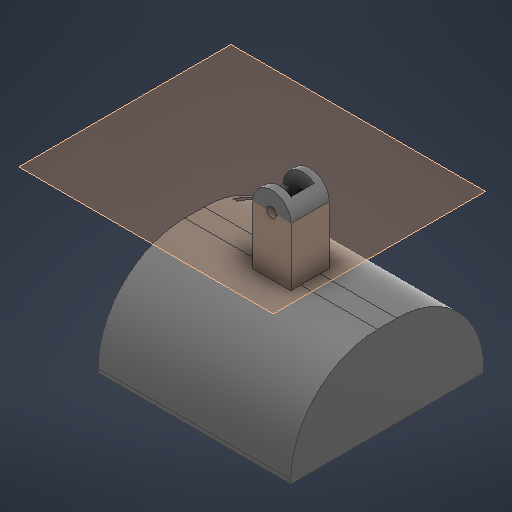
# Autodesk Inventor part: BuddyRobotBase
Saved by Autodesk Inventor 2026.2 (Build 302298000, 298)
## iProperties
Created: 2026-09-15
Part Number: BuddyRobotBase
Material: Generic
Document SubType Name: Modeling
Designer: User
Density: 1 g/cm^3
Appearance: Default
Author: User
Autodesk Inventor part; units mm, degrees
(part 1 of 2)
ref_plane "YZ Plane" through (0, 0, 0) normal (1, 0, 0) x (0, 1, 0)
ref_plane "XZ Plane" through (0, 0, 0) normal (0, 1, 0) x (-1, 0, 0)
ref_plane "XY Plane" through (0, 0, 0) normal (0, 0, 1) x (1, 0, 0)
sketch "Sketch1" plane through (0, 0, 0) normal (0, 1, 0) x (-1, 0, 0)
  line L0 (50, 50) -> (-50, 50)
  line L1 (-50, 50) -> (-50, -50)
  line L2 (-50, -50) -> (50, -50)
  line L3 (50, -50) -> (50, 50)
  line L4 (50, 50) -> (-50, -50) construction
  line L5 (-50, 50) -> (50, -50) construction
  point P0 (0, 0)
  dimension "d1" = 100
  dimension "d2" = 100
  constraints: 12 end point, 2 midpoint, 2 parallel, 1 horizontal, 1 perpendicular
  measures "d1" distance of L0.end L1.end
  measures "d2" distance of L0.start L0.end
extrude "Base" add sketch "Sketch1" along normal blind 2
sketch "Sketch2" plane through (50, 0, 50) normal (1, 0, 0) x (0, 0, -1)
  line L0 (0, 2) -> (100, 2) projected
  line L1 (0, 2) -> (100, 2)
  arc A0 (45, 47) -> (0, 2) centre (45, 2) ccw
  line L2 (0, 0) -> (0, 2) projected
  arc A1 (100, 2) -> (55, 47) centre (55, 2) ccw
  line L3 (100, 0) -> (100, 2) projected
  line L4 (45, 47) -> (55, 47)
  point P0 (50, 0)
  dimension "d6" = 10
  constraints: 4 end point, 4 point on circle, 3 tangent, 2 centre point, 1 collinear, 1 equal radius, 1 horizontal, 1 horizontal alignment
  measures "d6" distance of L4.start L4.end
extrude "Box" add sketch "Sketch2" against normal blind 100
shell "Shell" thickness 2 removed faces 1 at (-50, 15.6667, -1.6667)
sketch "Sketch4" plane through (50, 0, -50) normal (0, 0, -1) x (-1, 0, 0)
  line L0 (0, 2) -> (100, 2) projected
  line L1 (96, 2) -> (98, 2)
  line L2 (98, 2) -> (98, 45)
  line L3 (98, 45) -> (96, 45)
  line L4 (96, 45) -> (96, 2)
  line L5 (0, 47) -> (100, 47) projected
  line L6 (100, 2) -> (100, 47) projected
  point P0 (50, 0)
  dimension "d10" = 2
  dimension "d11" = 2
  dimension "d12" = 2
  constraints: 8 end point, 2 parallel, 1 horizontal, 1 perpendicular, 1 point on line
  measures "d10" distance between parallel lines of L5 L3
  measures "d11" distance between parallel lines of L6 L2
  measures "d12" distance between parallel lines of L2 L4
extrude "DoorSlot" cut sketch "Sketch4" against normal up to next
sketch "Sketch6" plane through (50, 47, 5) normal (0, 1, 0) x (1, 0, 0)
  line L0 (-40, 14.9) -> (-60, 14.9)
  line L1 (-60, 14.9) -> (-60, -4.9)
  line L2 (-60, -4.9) -> (-40, -4.9)
  line L3 (-40, -4.9) -> (-40, 14.9)
  line L4 (-40, 14.9) -> (-60, -4.9) construction
  line L5 (-60, 14.9) -> (-40, -4.9) construction
  line L6 (0, 10) -> (0, 0) projected
  point P0 (-50, 5)
  point P1 (-50, 5)
  dimension "d18" = 20
  dimension "d19" = 19.8
  dimension "d20" = 40
  constraints: 12 end point, 2 midpoint, 2 parallel, 1 coincident, 1 horizontal, 1 perpendicular
  measures "d18" distance of L0.start L0.end
  measures "d19" distance of L0.end L1.end
  measures "d20" distance between parallel lines of L6 L3
extrude "Extrusion5" add sketch "Sketch6" along normal blind 30 and the other way blind 0.5
sketch "Sketch7" plane through (-10, 46.7324, 9.9) normal (0, 0, 1) x (1, 0, 0)
  line L0 (0, 30.2676) -> (20, 30.2676) projected
  circle A0 centre (10, 30.2676) radius 10
  line L1 (20, 0) -> (20, 30.2676) projected
  point P0 (10, -46.7324)
  point P1 (20, 30.2676)
  point P2 (0, 30.2676)
  constraints: 1 centre point, 1 midpoint, 1 tangent
extrude "Extrusion6" add sketch "Sketch7" against normal blind 19.8 contours A0 L0 picked at (12.78, 34.8248)
sketch "Sketch8" plane through (-10, 46.7324, 9.9) normal (0, 0, 1) x (1, 0, 0)
  arc A0 (20, 30.2676) -> (0, 30.2676) centre (10, 30.2676) ccw projected
  circle A1 centre (10, 30.2676) radius 2.5
  point P0 (10, -46.7324)
  dimension "d27" = 5
  constraints: 1 centre point, 1 coincident
  measures "d27" diameter of A1
extrude "Extrusion7" cut sketch "Sketch8" against normal up to next
sketch "Sketch9" plane through (-50, 45, 5) normal (0, -1, 0) x (1, 0, 0)
  point P0 (50, -5)
ref_plane "Work Plane1" through (-10, 77, -9.9) normal (0, 1, 0) x (0, 0, 1)
sketch "Sketch10" plane through (-10, 77, -9.9) normal (0, 1, 0) x (0, 0, 1)
  line L0 (3.8, 16) -> (15.8, 16)
  line L1 (15.8, 16) -> (15.8, 4)
  line L2 (15.8, 4) -> (3.8, 4)
  line L3 (3.8, 4) -> (3.8, 16)
  line L4 (3.8, 16) -> (15.8, 4) construction
  line L5 (15.8, 16) -> (3.8, 4) construction
  line L6 (0, 0) -> (19.8, 0) projected
  line L7 (19.8, 0) -> (19.8, 20) projected
  point P0 (9.9, 10)
  point P1 (9.8, 10)
  dimension "d31" = 4
  dimension "d32" = 4
  dimension "d33" = 12
  dimension "d34" = 12
  constraints: 12 end point, 2 midpoint, 2 parallel, 1 horizontal, 1 perpendicular
  measures "d31" distance between parallel lines of L6 L2
  measures "d32" distance between parallel lines of L7 L1
  measures "d33" distance of L0.end L1.end
  measures "d34" distance of L1.end L2.end
extrude "Extrusion8" cut sketch "Sketch10" along normal blind 20 and the other way blind 40
sketch "Sketch11" plane through (-10, 47, -5) normal (-1, 0, 0) x (0, 0, 1)
  line L0 (-1.1, 38) -> (10.9, 38) projected
  line L1 (10.9, 32.5) -> (10.9, 27.5) projected
  line L2 (-1.1, 38) -> (10.9, 38)
  line L3 (10.9, 38) -> (10.9, 30)
  line L4 (10.9, 30) -> (-1.1, 30)
  line L5 (-1.1, 30) -> (-1.1, 38)
  point P0 (5, -47)
  point P1 (10.9, 32.5)
  point P2 (10.9, 38)
  constraints: 8 end point, 2 parallel, 1 horizontal, 1 midpoint, 1 perpendicular
extrude "Extrusion9" cut sketch "Sketch11" against normal up to next
sketch "Sketch12" plane through (48, 2, -48) normal (-1, 0, 0) x (0, 0, 1)
  arc A0 (43, 43) -> (0, 0) centre (43, 0) ccw projected
  line L0 (1.179, 10) -> (94.821, 10) construction
  line L1 (96, 0) -> (0, 0) projected
  arc A1 (96, 0) -> (53, 43) centre (53, 0) ccw projected
  spline S0 degree 2 poles (10.9376, 10.1) (10.3824, 9.8828) (9.5169, 9.8828) knots 0 0 0 1 1 1
  spline S1 degree 2 poles (9.5169, 9.8828) (9.41, 9.8828) (9.2203, 10.0828) (9.2203, 10.1897) knots 0 0 0 1 2 2 2
  line L2 (9.2203, 10.1897) -> (9.2203, 10.9103)
  spline S2 degree 2 poles (9.2203, 10.9103) (9.2203, 11.2621) (9.2652, 11.9172) knots 0 0 0 1 1 1
  spline S3 degree 2 poles (9.2652, 11.9172) (9.3134, 12.6241) (9.3169, 12.9414) knots 0 0 0 1 1 1
  spline S4 degree 2 poles (9.3169, 12.9414) (9.3169, 13.169) (9.3445, 13.6207) knots 0 0 0 1 1 1
  spline S5 degree 2 poles (9.3445, 13.6207) (9.3617, 13.7414) (9.4272, 13.7828) knots 0 0 0 1 1 1
  spline S6 degree 2 poles (9.4272, 13.7828) (9.7617, 13.8862) (10.1893, 13.8862) knots 0 0 0 1 1 1
  spline S7 degree 2 poles (10.1893, 13.8862) (10.6272, 13.8862) (11.0272, 13.5897) knots 0 0 0 1 1 1
  spline S8 degree 2 poles (11.0272, 13.5897) (11.4893, 13.2483) (11.4893, 12.7448) knots 0 0 0 1 1 1
  spline S9 degree 2 poles (11.4893, 12.7448) (11.4893, 12.1103) (10.9962, 11.7448) knots 0 0 0 1 1 1
  spline S10 degree 2 poles (10.9962, 11.7448) (11.3652, 11.5862) (11.7341, 11.2) (11.7341, 10.9724) knots 0 0 0 1 2 2 2
  spline S11 degree 2 poles (11.7341, 10.9724) (11.7341, 10.6724) (11.41, 10.3931) knots 0 0 0 1 1 1
  spline S12 degree 2 poles (11.41, 10.3931) (11.1858, 10.1966) (10.9376, 10.1) knots 0 0 0 1 1 1
  spline S13 degree 2 poles (10.1927, 13.3828) (9.9238, 13.3828) (9.8134, 13.3655) knots 0 0 0 1 1 1
  line L3 (9.8134, 13.3655) -> (9.81, 12.931)
  line L4 (9.81, 12.931) -> (9.7583, 11.9724)
  spline S14 degree 2 poles (9.7583, 11.9724) (10.11, 11.9414) (10.1341, 11.9448) knots 0 0 0 1 1 1
  spline S15 degree 2 poles (10.1341, 11.9448) (10.5065, 11.9759) (10.7445, 12.1793) knots 0 0 0 1 1 1
  spline S16 degree 2 poles (10.7445, 12.1793) (10.9996, 12.4) (10.9996, 12.7448) knots 0 0 0 1 1 1
  spline S17 degree 2 poles (10.9996, 12.7448) (10.9996, 12.9828) (10.4824, 13.3828) (10.1927, 13.3828) knots 0 0 0 1 2 2 2
  line L5 (10.4686, 11.4) -> (10.2065, 11.4414)
  spline S18 degree 2 poles (10.2065, 11.4414) (10.1755, 11.4414) (10.0445, 11.4345) (10.01, 11.4345) knots 0 0 0 1 2 2 2
  spline S19 degree 2 poles (10.01, 11.4345) (9.8755, 11.4345) (9.7238, 11.4552) knots 0 0 0 1 1 1
  spline S20 degree 2 poles (9.7238, 11.4552) (9.71, 11.1448) (9.71, 10.9) knots 0 0 0 1 1 1
  line L6 (9.71, 10.9) -> (9.71, 10.3897)
  spline S21 degree 2 poles (9.71, 10.3897) (10.3583, 10.4103) (10.7652, 10.5724) knots 0 0 0 1 1 1
  spline S22 degree 2 poles (10.7652, 10.5724) (10.9376, 10.6379) (11.0962, 10.7793) knots 0 0 0 1 1 1
  spline S23 degree 2 poles (11.0962, 10.7793) (11.2479, 10.9069) (11.2479, 10.9724) knots 0 0 0 1 1 1
  spline S24 degree 2 poles (11.2479, 10.9724) (11.2479, 11.0897) (10.9307, 11.2345) knots 0 0 0 1 1 1
  spline S25 degree 2 poles (10.9307, 11.2345) (10.6927, 11.3448) (10.4686, 11.4) knots 0 0 0 1 1 1
  spline S26 degree 2 poles (14.3031, 11.4448) (14.3031, 11.2655) (14.3065, 10.5552) (14.3065, 10.3759) knots 0 0 0 1 2 2 2
  spline S27 degree 2 poles (14.3065, 10.3759) (14.3065, 10.3241) (14.3238, 10.1) (14.3238, 10.0448) knots 0 0 0 1 2 2 2
  spline S28 degree 2 poles (14.3238, 10.0448) (14.3238, 9.9379) (14.179, 9.8034) (14.0755, 9.8034) knots 0 0 0 1 2 2 2
  spline S29 degree 2 poles (14.0755, 9.8034) (13.8858, 9.8034) (13.8341, 10.0379) knots 0 0 0 1 1 1
  spline S30 degree 2 poles (13.8341, 10.0379) (13.5238, 9.8759) (13.1203, 9.8759) knots 0 0 0 1 1 1
  spline S31 degree 2 poles (13.1203, 9.8759) (12.7962, 9.8759) (12.5824, 10.0207) knots 0 0 0 1 1 1
  spline S32 degree 2 poles (12.5824, 10.0207) (12.3479, 10.1793) (12.3031, 10.4828) knots 0 0 0 1 1 1
  spline S33 degree 2 poles (12.3031, 10.4828) (12.21, 11.1379) (12.21, 11.6517) knots 0 0 0 1 1 1
  spline S34 degree 2 poles (12.21, 11.6517) (12.21, 11.9897) (12.2824, 12.4241) knots 0 0 0 1 1 1
  spline S35 degree 2 poles (12.2824, 12.4241) (12.3169, 12.6379) (12.5169, 12.6379) knots 0 0 0 1 1 1
  spline S36 degree 2 poles (12.5169, 12.6379) (12.6238, 12.6379) (12.7652, 12.5034) (12.7652, 12.3966) knots 0 0 0 1 2 2 2
  spline S37 degree 2 poles (12.7652, 12.3966) (12.7652, 12.2828) (12.6962, 11.7828) (12.6962, 11.6517) knots 0 0 0 1 2 2 2
  spline S38 degree 2 poles (12.6962, 11.6517) (12.6962, 11.2379) (12.7514, 10.6483) (12.8031, 10.4724) knots 0 0 0 1 2 2 2
  spline S39 degree 2 poles (12.8031, 10.4724) (12.8858, 10.4276) (13.0445, 10.3793) (13.1203, 10.3793) knots 0 0 0 1 2 2 2
  spline S40 degree 2 poles (13.1203, 10.3793) (13.4548, 10.3793) (13.8238, 10.4862) knots 0 0 0 1 1 1
  line L7 (13.8238, 10.4862) -> (13.8203, 10.9862)
  line L8 (13.8203, 10.9862) -> (13.8169, 11.4655)
  spline S41 degree 2 poles (13.8169, 11.4655) (13.8169, 12) (13.8617, 12.3931) knots 0 0 0 1 1 1
  spline S42 degree 2 poles (13.8617, 12.3931) (13.8893, 12.6207) (14.0996, 12.6207) knots 0 0 0 1 1 1
  spline S43 degree 2 poles (14.0996, 12.6207) (14.2065, 12.6207) (14.3479, 12.4828) (14.3445, 12.3793) knots 0 0 0 1 2 2 2
  line L9 (14.3445, 12.3793) -> (14.3031, 11.4448)
  spline S44 degree 2 poles (17.1996, 12.1828) (17.1686, 11.8207) (17.1686, 11.4552) knots 0 0 0 1 1 1
  spline S45 degree 2 poles (17.1686, 11.4552) (17.1686, 10.631) (17.2445, 10.2103) knots 0 0 0 1 1 1
  spline S46 degree 2 poles (17.2445, 10.2103) (17.2514, 10.1759) (17.2514, 10.1552) knots 0 0 0 1 1 1
  spline S47 degree 2 poles (17.2514, 10.1552) (17.2514, 10.0552) (17.1134, 9.9276) (17.0203, 9.9276) knots 0 0 0 1 2 2 2
  spline S48 degree 2 poles (17.0203, 9.9276) (16.8686, 9.9276) (16.7962, 10.1517) knots 0 0 0 1 1 1
  spline S49 degree 2 poles (16.7962, 10.1517) (16.6169, 10.0207) (16.2341, 9.8862) (16.0272, 9.8862) knots 0 0 0 1 2 2 2
  spline S50 degree 2 poles (16.0272, 9.8862) (15.5134, 9.8862) (15.179, 10.2276) knots 0 0 0 1 1 1
  spline S51 degree 2 poles (15.179, 10.2276) (14.8307, 10.5759) (14.8307, 11.1241) knots 0 0 0 1 1 1
  spline S52 degree 2 poles (14.8307, 11.1241) (14.8307, 11.7828) (15.5307, 12.5793) (16.0893, 12.5793) knots 0 0 0 1 2 2 2
  spline S53 degree 2 poles (16.0893, 12.5793) (16.3755, 12.5793) (16.5341, 12.4897) knots 0 0 0 1 1 1
  line L10 (16.5341, 12.4897) -> (16.7652, 12.3207)
  spline S54 degree 2 poles (16.7652, 12.3207) (16.7996, 13.3621) (16.8479, 13.7207) knots 0 0 0 1 1 1
  spline S55 degree 2 poles (16.8479, 13.7207) (16.879, 13.9414) (17.0721, 13.9414) knots 0 0 0 1 1 1
  spline S56 degree 2 poles (17.0721, 13.9414) (17.2962, 13.9414) (17.2962, 13.7) knots 0 0 0 1 1 1
  spline S57 degree 2 poles (17.2962, 13.7) (17.2962, 13.3586) (17.1996, 12.1828) knots 0 0 0 1 1 1
  spline S58 degree 2 poles (16.0996, 12.1207) (15.6858, 12.1207) (15.2686, 11.6276) (15.2686, 11.1345) knots 0 0 0 1 2 2 2
  spline S59 degree 2 poles (15.2686, 11.1345) (15.2686, 10.8138) (15.7203, 10.3552) (16.0272, 10.3552) knots 0 0 0 1 2 2 2
  spline S60 degree 2 poles (16.0272, 10.3552) (16.2341, 10.3552) (16.379, 10.431) knots 0 0 0 1 1 1
  spline S61 degree 2 poles (16.379, 10.431) (16.4617, 10.4759) (16.6514, 10.6379) knots 0 0 0 1 1 1
  spline S62 degree 2 poles (16.6514, 10.6379) (16.6893, 10.669) (16.7238, 10.7138) knots 0 0 0 1 1 1
  line L11 (16.7238, 10.7138) -> (16.7169, 11.1414)
  line L12 (16.7169, 11.1414) -> (16.7203, 11.4276)
  line L13 (16.7203, 11.4276) -> (16.7238, 11.7207)
  spline S63 degree 2 poles (16.7238, 11.7207) (16.6307, 11.9207) (16.3169, 12.1207) (16.0996, 12.1207) knots 0 0 0 1 2 2 2
  spline S64 degree 2 poles (20.1755, 12.1828) (20.1445, 11.8207) (20.1445, 11.4552) knots 0 0 0 1 1 1
  spline S65 degree 2 poles (20.1445, 11.4552) (20.1445, 10.631) (20.2203, 10.2103) knots 0 0 0 1 1 1
  spline S66 degree 2 poles (20.2203, 10.2103) (20.2272, 10.1759) (20.2272, 10.1552) knots 0 0 0 1 1 1
  spline S67 degree 2 poles (20.2272, 10.1552) (20.2272, 10.0552) (20.0893, 9.9276) (19.9962, 9.9276) knots 0 0 0 1 2 2 2
  spline S68 degree 2 poles (19.9962, 9.9276) (19.8445, 9.9276) (19.7721, 10.1517) knots 0 0 0 1 1 1
  spline S69 degree 2 poles (19.7721, 10.1517) (19.5927, 10.0207) (19.21, 9.8862) (19.0031, 9.8862) knots 0 0 0 1 2 2 2
  spline S70 degree 2 poles (19.0031, 9.8862) (18.4893, 9.8862) (18.1548, 10.2276) knots 0 0 0 1 1 1
  spline S71 degree 2 poles (18.1548, 10.2276) (17.8065, 10.5759) (17.8065, 11.1241) knots 0 0 0 1 1 1
  spline S72 degree 2 poles (17.8065, 11.1241) (17.8065, 11.7828) (18.5065, 12.5793) (19.0652, 12.5793) knots 0 0 0 1 2 2 2
  spline S73 degree 2 poles (19.0652, 12.5793) (19.3514, 12.5793) (19.51, 12.4897) knots 0 0 0 1 1 1
  line L14 (19.51, 12.4897) -> (19.741, 12.3207)
  spline S74 degree 2 poles (19.741, 12.3207) (19.7755, 13.3621) (19.8238, 13.7207) knots 0 0 0 1 1 1
  spline S75 degree 2 poles (19.8238, 13.7207) (19.8548, 13.9414) (20.0479, 13.9414) knots 0 0 0 1 1 1
  spline S76 degree 2 poles (20.0479, 13.9414) (20.2721, 13.9414) (20.2721, 13.7) knots 0 0 0 1 1 1
  spline S77 degree 2 poles (20.2721, 13.7) (20.2721, 13.3586) (20.1755, 12.1828) knots 0 0 0 1 1 1
  spline S78 degree 2 poles (19.0755, 12.1207) (18.6617, 12.1207) (18.2445, 11.6276) (18.2445, 11.1345) knots 0 0 0 1 2 2 2
  spline S79 degree 2 poles (18.2445, 11.1345) (18.2445, 10.8138) (18.6962, 10.3552) (19.0031, 10.3552) knots 0 0 0 1 2 2 2
  spline S80 degree 2 poles (19.0031, 10.3552) (19.21, 10.3552) (19.3548, 10.431) knots 0 0 0 1 1 1
  spline S81 degree 2 poles (19.3548, 10.431) (19.4376, 10.4759) (19.6272, 10.6379) knots 0 0 0 1 1 1
  spline S82 degree 2 poles (19.6272, 10.6379) (19.6652, 10.669) (19.6996, 10.7138) knots 0 0 0 1 1 1
  line L15 (19.6996, 10.7138) -> (19.6927, 11.1414)
  line L16 (19.6927, 11.1414) -> (19.6962, 11.4276)
  line L17 (19.6962, 11.4276) -> (19.6996, 11.7207)
  spline S83 degree 2 poles (19.6996, 11.7207) (19.6065, 11.9207) (19.2927, 12.1207) (19.0755, 12.1207) knots 0 0 0 1 2 2 2
  line L18 (23.0272, 12.2069) -> (22.1721, 10.3552)
  spline S84 degree 2 poles (22.1721, 10.3552) (21.8548, 9.6793) (21.6858, 9.2241) knots 0 0 0 1 1 1
  line L19 (21.6858, 9.2241) -> (21.5238, 8.7448)
  spline S85 degree 2 poles (21.5238, 8.7448) (21.4583, 8.569) (21.3031, 8.569) knots 0 0 0 1 1 1
  spline S86 degree 2 poles (21.3031, 8.569) (21.1996, 8.569) (21.0479, 8.7034) (21.0479, 8.8069) knots 0 0 0 1 2 2 2
  spline S87 degree 2 poles (21.0479, 8.8069) (21.0479, 9.0517) (21.5824, 10.2379) knots 0 0 0 1 1 1
  line L20 (21.5824, 10.2379) -> (20.6962, 11.9414)
  line L21 (20.6962, 11.9414) -> (20.5824, 12.1207)
  spline S88 degree 2 poles (20.5824, 12.1207) (20.5169, 12.2345) (20.5169, 12.3138) knots 0 0 0 1 1 1
  spline S89 degree 2 poles (20.5169, 12.3138) (20.5169, 12.4138) (20.6721, 12.569) (20.7686, 12.569) knots 0 0 0 1 2 2 2
  spline S90 degree 2 poles (20.7686, 12.569) (20.8824, 12.569) (20.9445, 12.4793) knots 0 0 0 1 1 1
  spline S91 degree 2 poles (20.9445, 12.4793) (21.3652, 11.8931) (21.8479, 10.8103) knots 0 0 0 1 1 1
  line L22 (21.8479, 10.8103) -> (22.2169, 11.6724)
  spline S92 degree 2 poles (22.2169, 11.6724) (22.4134, 12.1138) (22.5962, 12.4345) knots 0 0 0 1 1 1
  spline S93 degree 2 poles (22.5962, 12.4345) (22.6755, 12.5724) (22.8031, 12.5724) knots 0 0 0 1 1 1
  spline S94 degree 2 poles (22.8031, 12.5724) (22.9031, 12.5724) (23.0583, 12.4276) (23.0583, 12.331) knots 0 0 0 1 2 2 2
  spline S95 degree 2 poles (23.0583, 12.331) (23.0583, 12.2759) (23.0272, 12.2069) knots 0 0 0 1 1 1
  spline S96 degree 2 poles (26.8686, 10.1) (26.3134, 9.8828) (25.4479, 9.8828) knots 0 0 0 1 1 1
  spline S97 degree 2 poles (25.4479, 9.8828) (25.341, 9.8828) (25.1514, 10.0828) (25.1514, 10.1897) knots 0 0 0 1 2 2 2
  line L23 (25.1514, 10.1897) -> (25.1514, 10.9103)
  spline S98 degree 2 poles (25.1514, 10.9103) (25.1514, 11.2621) (25.1962, 11.9172) knots 0 0 0 1 1 1
  spline S99 degree 2 poles (25.1962, 11.9172) (25.2445, 12.6241) (25.2479, 12.9414) knots 0 0 0 1 1 1
  spline S100 degree 2 poles (25.2479, 12.9414) (25.2479, 13.169) (25.2755, 13.6207) knots 0 0 0 1 1 1
  spline S101 degree 2 poles (25.2755, 13.6207) (25.2927, 13.7414) (25.3583, 13.7828) knots 0 0 0 1 1 1
  spline S102 degree 2 poles (25.3583, 13.7828) (25.6927, 13.8862) (26.1203, 13.8862) knots 0 0 0 1 1 1
  spline S103 degree 2 poles (26.1203, 13.8862) (26.5583, 13.8862) (26.9583, 13.5897) knots 0 0 0 1 1 1
  spline S104 degree 2 poles (26.9583, 13.5897) (27.4203, 13.2483) (27.4203, 12.7448) knots 0 0 0 1 1 1
  spline S105 degree 2 poles (27.4203, 12.7448) (27.4203, 12.1103) (26.9272, 11.7448) knots 0 0 0 1 1 1
  spline S106 degree 2 poles (26.9272, 11.7448) (27.2962, 11.5862) (27.6652, 11.2) (27.6652, 10.9724) knots 0 0 0 1 2 2 2
  spline S107 degree 2 poles (27.6652, 10.9724) (27.6652, 10.6724) (27.341, 10.3931) knots 0 0 0 1 1 1
  spline S108 degree 2 poles (27.341, 10.3931) (27.1169, 10.1966) (26.8686, 10.1) knots 0 0 0 1 1 1
  spline S109 degree 2 poles (26.1238, 13.3828) (25.8548, 13.3828) (25.7445, 13.3655) knots 0 0 0 1 1 1
  line L24 (25.7445, 13.3655) -> (25.741, 12.931)
  line L25 (25.741, 12.931) -> (25.6893, 11.9724)
  spline S110 degree 2 poles (25.6893, 11.9724) (26.041, 11.9414) (26.0652, 11.9448) knots 0 0 0 1 1 1
  spline S111 degree 2 poles (26.0652, 11.9448) (26.4376, 11.9759) (26.6755, 12.1793) knots 0 0 0 1 1 1
  spline S112 degree 2 poles (26.6755, 12.1793) (26.9307, 12.4) (26.9307, 12.7448) knots 0 0 0 1 1 1
  spline S113 degree 2 poles (26.9307, 12.7448) (26.9307, 12.9828) (26.4134, 13.3828) (26.1238, 13.3828) knots 0 0 0 1 2 2 2
  line L26 (26.3996, 11.4) -> (26.1376, 11.4414)
  spline S114 degree 2 poles (26.1376, 11.4414) (26.1065, 11.4414) (25.9755, 11.4345) (25.941, 11.4345) knots 0 0 0 1 2 2 2
  spline S115 degree 2 poles (25.941, 11.4345) (25.8065, 11.4345) (25.6548, 11.4552) knots 0 0 0 1 1 1
  spline S116 degree 2 poles (25.6548, 11.4552) (25.641, 11.1448) (25.641, 10.9) knots 0 0 0 1 1 1
  line L27 (25.641, 10.9) -> (25.641, 10.3897)
  spline S117 degree 2 poles (25.641, 10.3897) (26.2893, 10.4103) (26.6962, 10.5724) knots 0 0 0 1 1 1
  spline S118 degree 2 poles (26.6962, 10.5724) (26.8686, 10.6379) (27.0272, 10.7793) knots 0 0 0 1 1 1
  spline S119 degree 2 poles (27.0272, 10.7793) (27.179, 10.9069) (27.179, 10.9724) knots 0 0 0 1 1 1
  spline S120 degree 2 poles (27.179, 10.9724) (27.179, 11.0897) (26.8617, 11.2345) knots 0 0 0 1 1 1
  spline S121 degree 2 poles (26.8617, 11.2345) (26.6238, 11.3448) (26.3996, 11.4) knots 0 0 0 1 1 1
  spline S122 degree 2 poles (29.1479, 9.8552) (28.7341, 9.8552) (28.4341, 10.1621) knots 0 0 0 1 1 1
  spline S123 degree 2 poles (28.4341, 10.1621) (28.0996, 10.5034) (28.0824, 11.0793) knots 0 0 0 1 1 1
  spline S124 degree 2 poles (28.0824, 11.0793) (28.0686, 11.6379) (28.3652, 12.0621) knots 0 0 0 1 1 1
  spline S125 degree 2 poles (28.3652, 12.0621) (28.71, 12.5655) (29.3272, 12.5655) knots 0 0 0 1 1 1
  spline S126 degree 2 poles (29.3272, 12.5655) (29.8238, 12.5655) (30.0755, 12.1138) knots 0 0 0 1 1 1
  spline S127 degree 2 poles (30.0755, 12.1138) (30.279, 11.7483) (30.2721, 11.231) knots 0 0 0 1 1 1
  spline S128 degree 2 poles (30.2721, 11.231) (30.2652, 10.6828) (29.9859, 10.2966) knots 0 0 0 1 1 1
  spline S129 degree 2 poles (29.9859, 10.2966) (29.6686, 9.8552) (29.1479, 9.8552) knots 0 0 0 1 1 1
  spline S130 degree 2 poles (29.2962, 12.0621) (28.9341, 12.0655) (28.7307, 11.7172) knots 0 0 0 1 1 1
  spline S131 degree 2 poles (28.7307, 11.7172) (28.5686, 11.4379) (28.5686, 11.0793) knots 0 0 0 1 1 1
  spline S132 degree 2 poles (28.5686, 11.0793) (28.5686, 10.7207) (28.7652, 10.5207) knots 0 0 0 1 1 1
  spline S133 degree 2 poles (28.7652, 10.5207) (28.9272, 10.3552) (29.1479, 10.3552) knots 0 0 0 1 1 1
  spline S134 degree 2 poles (29.1479, 10.3552) (29.4065, 10.3552) (29.5893, 10.5414) knots 0 0 0 1 1 1
  spline S135 degree 2 poles (29.5893, 10.5414) (29.7996, 10.7517) (29.8134, 11.1034) knots 0 0 0 1 1 1
  spline S136 degree 2 poles (29.8134, 11.1034) (29.8479, 12.0586) (29.2962, 12.0621) knots 0 0 0 1 1 1
  spline S137 degree 2 poles (32.5376, 12.1069) (32.4859, 12.1069) (32.3445, 12.1172) (32.2927, 12.1172) knots 0 0 0 1 2 2 2
  spline S138 degree 2 poles (32.2927, 12.1172) (32.2341, 12.1172) (31.9548, 12.0793) knots 0 0 0 1 1 1
  line L28 (31.9548, 12.0793) -> (31.9996, 10.6172)
  line L29 (31.9996, 10.6172) -> (32.0031, 10.5103)
  line L30 (32.0031, 10.5103) -> (32.0065, 10.3828)
  spline S139 degree 2 poles (32.0065, 10.3828) (32.0169, 9.8414) (31.7479, 9.8414) knots 0 0 0 1 1 1
  spline S140 degree 2 poles (31.7479, 9.8414) (31.6479, 9.8414) (31.5031, 9.969) (31.5031, 10.0655) knots 0 0 0 1 2 2 2
  spline S141 degree 2 poles (31.5031, 10.0655) (31.5031, 10.1621) (31.5169, 10.5379) (31.5169, 10.631) knots 0 0 0 1 2 2 2
  line L31 (31.5169, 10.631) -> (31.4686, 12.0759)
  spline S142 degree 2 poles (31.4686, 12.0759) (31.2893, 12.0828) (30.9203, 12.1172) knots 0 0 0 1 1 1
  spline S143 degree 2 poles (30.9203, 12.1172) (30.6996, 12.1483) (30.6996, 12.3621) knots 0 0 0 1 1 1
  spline S144 degree 2 poles (30.6996, 12.3621) (30.6996, 12.4724) (30.8341, 12.6138) (30.9376, 12.6138) knots 0 0 0 1 2 2 2
  line L32 (30.9376, 12.6138) -> (31.4548, 12.5724)
  spline S145 degree 2 poles (31.4548, 12.5724) (31.4548, 12.7) (31.4341, 13.1207) (31.4341, 13.2138) knots 0 0 0 1 2 2 2
  spline S146 degree 2 poles (31.4341, 13.2138) (31.4341, 13.3207) (31.5755, 13.4552) (31.679, 13.4552) knots 0 0 0 1 2 2 2
  spline S147 degree 2 poles (31.679, 13.4552) (31.9031, 13.4552) (31.941, 13.0931) knots 0 0 0 1 1 1
  spline S148 degree 2 poles (31.941, 13.0931) (31.9479, 13) (31.9479, 12.8724) knots 0 0 0 1 1 1
  line L33 (31.9479, 12.8724) -> (31.9445, 12.7276)
  line L34 (31.9445, 12.7276) -> (31.941, 12.5759)
  spline S149 degree 2 poles (31.941, 12.5759) (32.2479, 12.6138) (32.2927, 12.6138) knots 0 0 0 1 1 1
  spline S150 degree 2 poles (32.2927, 12.6138) (32.5479, 12.6138) (32.6272, 12.5897) knots 0 0 0 1 1 1
  spline S151 degree 2 poles (32.6272, 12.5897) (32.779, 12.5414) (32.779, 12.3586) knots 0 0 0 1 1 1
  spline S152 degree 2 poles (32.779, 12.3586) (32.779, 12.2483) (32.6445, 12.1069) (32.5376, 12.1069) knots 0 0 0 1 2 2 2
  spline S153 degree 2 poles (37.6686, 13.3897) (37.5134, 13.1621) (37.4169, 12.9103) knots 0 0 0 1 1 1
  line L35 (37.4169, 12.9103) -> (37.2307, 12.369)
  line L36 (37.2307, 12.369) -> (36.5652, 10.569)
  spline S154 degree 2 poles (36.5652, 10.569) (36.4479, 10.2552) (36.2927, 9.9517) knots 0 0 0 1 1 1
  spline S155 degree 2 poles (36.2927, 9.9517) (36.2134, 9.8034) (36.0686, 9.8034) knots 0 0 0 1 1 1
  spline S156 degree 2 poles (36.0686, 9.8034) (35.879, 9.8034) (35.8031, 9.9966) knots 0 0 0 1 1 1
  spline S157 degree 2 poles (35.8031, 9.9966) (35.5031, 10.7483) (35.1376, 12.1586) knots 0 0 0 1 1 1
  line L37 (35.1376, 12.1586) -> (34.941, 12.8414)
  spline S158 degree 2 poles (34.941, 12.8414) (34.7962, 13.3552) (34.7962, 13.5138) knots 0 0 0 1 1 1
  spline S159 degree 2 poles (34.7962, 13.5138) (34.7962, 13.6241) (34.8755, 13.6966) knots 0 0 0 1 1 1
  spline S160 degree 2 poles (34.8755, 13.6966) (34.9479, 13.7621) (35.0479, 13.7621) knots 0 0 0 1 1 1
  spline S161 degree 2 poles (35.0479, 13.7621) (35.2376, 13.7621) (35.2893, 13.5586) knots 0 0 0 1 1 1
  line L38 (35.2893, 13.5586) -> (35.3824, 13.1276)
  line L39 (35.3824, 13.1276) -> (35.6203, 12.2897)
  spline S162 degree 2 poles (35.6203, 12.2897) (35.8548, 11.369) (36.0824, 10.7034) knots 0 0 0 1 1 1
  line L40 (36.0824, 10.7034) -> (36.0962, 10.7448)
  line L41 (36.0962, 10.7448) -> (36.7583, 12.5379)
  line L42 (36.7583, 12.5379) -> (36.9686, 13.1448)
  spline S163 degree 2 poles (36.9686, 13.1448) (37.11, 13.5103) (37.2686, 13.6966) knots 0 0 0 1 1 1
  spline S164 degree 2 poles (37.2686, 13.6966) (37.3514, 13.7966) (37.4617, 13.7966) knots 0 0 0 1 1 1
  spline S165 degree 2 poles (37.4617, 13.7966) (37.5617, 13.7966) (37.7169, 13.6448) (37.7169, 13.5379) knots 0 0 0 1 2 2 2
  spline S166 degree 2 poles (37.7169, 13.5379) (37.7169, 13.4655) (37.6686, 13.3897) knots 0 0 0 1 1 1
  line L43 (39.4721, 9.9966) -> (38.9824, 9.9966)
  line L44 (38.9824, 9.9966) -> (38.4927, 10)
  spline S167 degree 2 poles (38.4927, 10) (38.3203, 10) (38.2514, 10.0207) knots 0 0 0 1 1 1
  spline S168 degree 2 poles (38.2514, 10.0207) (38.1238, 10.0655) (38.1238, 10.2103) knots 0 0 0 1 1 1
  spline S169 degree 2 poles (38.1238, 10.2103) (38.1238, 10.4586) (38.51, 10.4586) knots 0 0 0 1 1 1
  line L45 (38.51, 10.4586) -> (38.6307, 10.4552)
  line L46 (38.6307, 10.4552) -> (38.7307, 10.4517)
  spline S170 degree 2 poles (38.7307, 10.4517) (38.7307, 10.569) (38.6893, 11.0345) (38.6893, 11.1517) knots 0 0 0 1 2 2 2
  spline S171 degree 2 poles (38.6893, 11.1517) (38.6893, 11.4655) (38.7445, 12.1069) knots 0 0 0 1 1 1
  spline S172 degree 2 poles (38.7445, 12.1069) (38.7996, 12.7345) (38.7962, 13.0621) knots 0 0 0 1 1 1
  spline S173 degree 2 poles (38.7962, 13.0621) (38.4652, 12.8034) (38.3755, 12.8034) knots 0 0 0 1 1 1
  spline S174 degree 2 poles (38.3755, 12.8034) (38.2755, 12.8034) (38.1307, 12.9517) (38.1307, 13.0483) knots 0 0 0 1 2 2 2
  spline S175 degree 2 poles (38.1307, 13.0483) (38.1307, 13.1655) (38.3445, 13.331) knots 0 0 0 1 1 1
  spline S176 degree 2 poles (38.3445, 13.331) (38.4755, 13.4276) (38.7203, 13.6345) knots 0 0 0 1 1 1
  spline S177 degree 2 poles (38.7203, 13.6345) (38.941, 13.8552) (39.1376, 13.8552) knots 0 0 0 1 1 1
  spline S178 degree 2 poles (39.1376, 13.8552) (39.3031, 13.8552) (39.3031, 13.6655) knots 0 0 0 1 1 1
  spline S179 degree 2 poles (39.3031, 13.6655) (39.3031, 13.6069) (39.2721, 13.3828) (39.2721, 13.3241) knots 0 0 0 1 2 2 2
  spline S180 degree 2 poles (39.2721, 13.3241) (39.2721, 13.2448) (39.2893, 12.9138) (39.2893, 12.831) knots 0 0 0 1 2 2 2
  spline S181 degree 2 poles (39.2893, 12.831) (39.2893, 12.5483) (39.1721, 11.431) (39.1721, 11.1517) knots 0 0 0 1 2 2 2
  spline S182 degree 2 poles (39.1721, 11.1517) (39.1721, 11.0069) (39.21, 10.5966) (39.2134, 10.4655) knots 0 0 0 1 2 2 2
  line L47 (39.2134, 10.4655) -> (39.4721, 10.469)
  spline S183 degree 2 poles (39.4721, 10.469) (39.579, 10.469) (39.7134, 10.3345) (39.7134, 10.2345) knots 0 0 0 1 2 2 2
  spline S184 degree 2 poles (39.7134, 10.2345) (39.7134, 10.131) (39.579, 9.9966) (39.4721, 9.9966) knots 0 0 0 1 2 2 2
  spline S185 degree 2 poles (40.6721, 9.769) (40.5445, 9.769) (40.3652, 9.9483) (40.3652, 10.0759) knots 0 0 0 1 2 2 2
  spline S186 degree 2 poles (40.3652, 10.0759) (40.3652, 10.2034) (40.5445, 10.3828) (40.6721, 10.3828) knots 0 0 0 1 2 2 2
  spline S187 degree 2 poles (40.6721, 10.3828) (40.7996, 10.3828) (40.979, 10.2034) (40.979, 10.0759) knots 0 0 0 1 2 2 2
  spline S188 degree 2 poles (40.979, 10.0759) (40.979, 9.9483) (40.7996, 9.769) (40.6721, 9.769) knots 0 0 0 1 2 2 2
  spline S189 degree 2 poles (42.7859, 9.9034) (42.0341, 9.9034) (41.6893, 10.5897) knots 0 0 0 1 1 1
  spline S190 degree 2 poles (41.6893, 10.5897) (41.4272, 11.1207) (41.4272, 11.969) knots 0 0 0 1 1 1
  spline S191 degree 2 poles (41.4272, 11.969) (41.4272, 12.6862) (41.7686, 13.2207) knots 0 0 0 1 1 1
  spline S192 degree 2 poles (41.7686, 13.2207) (42.1721, 13.8448) (42.8617, 13.8448) knots 0 0 0 1 1 1
  spline S193 degree 2 poles (42.8617, 13.8448) (43.5134, 13.8448) (43.8755, 13.2897) knots 0 0 0 1 1 1
  spline S194 degree 2 poles (43.8755, 13.2897) (44.1893, 12.8103) (44.1893, 12.1207) knots 0 0 0 1 1 1
  spline S195 degree 2 poles (44.1893, 12.1207) (44.1893, 11.0138) (43.4893, 9.9034) (42.7859, 9.9034) knots 0 0 0 1 2 2 2
  spline S196 degree 2 poles (42.8617, 13.369) (42.3996, 13.369) (42.1307, 12.9) knots 0 0 0 1 1 1
  spline S197 degree 2 poles (42.1307, 12.9) (41.9065, 12.5103) (41.9065, 12.0103) knots 0 0 0 1 1 1
  spline S198 degree 2 poles (41.9065, 12.0103) (41.9065, 11.1966) (42.3479, 10.3793) (42.7859, 10.3793) knots 0 0 0 1 2 2 2
  spline S199 degree 2 poles (42.7859, 10.3793) (43.31, 10.3793) (43.5376, 10.9793) knots 0 0 0 1 1 1
  spline S200 degree 2 poles (43.5376, 10.9793) (43.6962, 11.3931) (43.6962, 12.031) knots 0 0 0 1 1 1
  spline S201 degree 2 poles (43.6962, 12.031) (43.6962, 12.7) (43.279, 13.369) (42.8617, 13.369) knots 0 0 0 1 2 2 2
  spline S202 degree 2 poles (47.5583, 11.1759) (47.2238, 11.1414) (46.3617, 11.1414) knots 0 0 0 1 1 1
  spline S203 degree 2 poles (46.3617, 11.1414) (46.1548, 11.1414) (46.1548, 11.3345) knots 0 0 0 1 1 1
  spline S204 degree 2 poles (46.1548, 11.3345) (46.1548, 11.5276) (46.3617, 11.5276) knots 0 0 0 1 1 1
  spline S205 degree 2 poles (46.3617, 11.5276) (46.5583, 11.5276) (47.341, 11.5621) (47.5341, 11.5621) knots 0 0 0 1 2 2 2
  spline S206 degree 2 poles (47.5341, 11.5621) (47.7548, 11.5621) (47.7548, 11.369) knots 0 0 0 1 1 1
  spline S207 degree 2 poles (47.7548, 11.369) (47.7548, 11.2) (47.5583, 11.1759) knots 0 0 0 1 1 1
  spline S208 degree 2 poles (52.8721, 13.1241) (52.6893, 13.1241) (52.3065, 13.1552) knots 0 0 0 1 1 1
  spline S209 degree 2 poles (52.3065, 13.1552) (51.9376, 13.1828) (51.7445, 13.1793) knots 0 0 0 1 1 1
  line L48 (51.7445, 13.1793) -> (51.5686, 13.1793)
  spline S210 degree 2 poles (51.5686, 13.1793) (51.5755, 12.8379) (51.6341, 12.069) knots 0 0 0 1 1 1
  spline S211 degree 2 poles (51.6341, 12.069) (51.6893, 11.3552) (51.6893, 10.9586) knots 0 0 0 1 1 1
  spline S212 degree 2 poles (51.6893, 10.9586) (51.6893, 10.8724) (51.7238, 10.5207) (51.7238, 10.431) knots 0 0 0 1 2 2 2
  spline S213 degree 2 poles (51.7238, 10.431) (51.7238, 10.2655) (51.6686, 10.1414) knots 0 0 0 1 1 1
  spline S214 degree 2 poles (51.6686, 10.1414) (51.5996, 9.9793) (51.4548, 9.9793) knots 0 0 0 1 1 1
  spline S215 degree 2 poles (51.4548, 9.9793) (51.3548, 9.9793) (51.1962, 10.1172) (51.1962, 10.2276) knots 0 0 0 1 2 2 2
  spline S216 degree 2 poles (51.1962, 10.2276) (51.1962, 10.2655) (51.2203, 10.4138) (51.2203, 10.4483) knots 0 0 0 1 2 2 2
  spline S217 degree 2 poles (51.2203, 10.4483) (51.2203, 10.5724) (51.1893, 11.0552) (51.1893, 11.1793) knots 0 0 0 1 2 2 2
  spline S218 degree 2 poles (51.1893, 11.1793) (51.1893, 11.5345) (51.1307, 12.1759) knots 0 0 0 1 1 1
  spline S219 degree 2 poles (51.1307, 12.1759) (51.0721, 12.8655) (51.0652, 13.169) knots 0 0 0 1 1 1
  line L49 (51.0652, 13.169) -> (50.841, 13.1655)
  spline S220 degree 2 poles (50.841, 13.1655) (50.2996, 13.1655) (49.9893, 13.2448) knots 0 0 0 1 1 1
  spline S221 degree 2 poles (49.9893, 13.2448) (49.7893, 13.2966) (49.7893, 13.4897) knots 0 0 0 1 1 1
  spline S222 degree 2 poles (49.7893, 13.4897) (49.7893, 13.5931) (49.8548, 13.669) knots 0 0 0 1 1 1
  spline S223 degree 2 poles (49.8548, 13.669) (49.9272, 13.7552) (50.0445, 13.7483) knots 0 0 0 1 1 1
  spline S224 degree 2 poles (50.0445, 13.7483) (50.1307, 13.7448) (50.441, 13.7034) knots 0 0 0 1 1 1
  spline S225 degree 2 poles (50.441, 13.7034) (50.6859, 13.6724) (50.841, 13.6724) knots 0 0 0 1 1 1
  spline S226 degree 2 poles (50.841, 13.6724) (50.9893, 13.6724) (51.5927, 13.6862) (51.741, 13.6862) knots 0 0 0 1 2 2 2
  spline S227 degree 2 poles (51.741, 13.6862) (51.9307, 13.6862) (52.679, 13.631) (52.8721, 13.631) knots 0 0 0 1 2 2 2
  spline S228 degree 2 poles (52.8721, 13.631) (52.9755, 13.631) (53.1203, 13.4862) (53.1203, 13.3759) knots 0 0 0 1 2 2 2
  spline S229 degree 2 poles (53.1203, 13.3759) (53.1203, 13.2724) (52.9755, 13.1241) (52.8721, 13.1241) knots 0 0 0 1 2 2 2
  spline S230 degree 2 poles (55.2203, 9.8345) (55.1755, 9.8345) (55.0514, 9.9448) knots 0 0 0 1 1 1
  spline S231 degree 2 poles (55.0514, 9.9448) (54.941, 10.0448) (54.8859, 10.1241) knots 0 0 0 1 1 1
  spline S232 degree 2 poles (54.8859, 10.1241) (54.6479, 9.9966) (54.2859, 9.8655) (54.1652, 9.8655) knots 0 0 0 1 2 2 2
  spline S233 degree 2 poles (54.1652, 9.8655) (53.5859, 9.8655) (53.3203, 10.1931) knots 0 0 0 1 1 1
  spline S234 degree 2 poles (53.3203, 10.1931) (53.0721, 10.5) (53.0721, 11.131) knots 0 0 0 1 1 1
  spline S235 degree 2 poles (53.0721, 11.131) (53.0721, 11.731) (53.8962, 12.5828) (54.4686, 12.5828) knots 0 0 0 1 2 2 2
  spline S236 degree 2 poles (54.4686, 12.5828) (54.6824, 12.5828) (54.9514, 12.4724) knots 0 0 0 1 1 1
  spline S237 degree 2 poles (54.9514, 12.4724) (55.2859, 12.331) (55.2859, 12.1379) knots 0 0 0 1 1 1
  spline S238 degree 2 poles (55.2859, 12.1379) (55.2859, 12.069) (55.2376, 12.0172) knots 0 0 0 1 1 1
  spline S239 degree 2 poles (55.2376, 12.0172) (55.2134, 11.9241) (55.1859, 11.4931) (55.1824, 11.1552) knots 0 0 0 1 2 2 2
  spline S240 degree 2 poles (55.1824, 11.1552) (55.179, 10.8483) (55.2238, 10.6724) knots 0 0 0 1 1 1
  spline S241 degree 2 poles (55.2238, 10.6724) (55.2479, 10.5621) (55.379, 10.2345) knots 0 0 0 1 1 1
  spline S242 degree 2 poles (55.379, 10.2345) (55.3962, 10.1897) (55.4376, 10.1034) knots 0 0 0 1 1 1
  line L50 (55.4376, 10.1034) -> (55.4514, 10.0621)
  spline S243 degree 2 poles (55.4514, 10.0621) (55.4514, 9.9621) (55.3134, 9.8345) (55.2203, 9.8345) knots 0 0 0 1 2 2 2
  spline S244 degree 2 poles (54.7065, 11.5552) (54.7065, 11.6621) (54.7341, 11.9138) (54.7617, 12.0517) knots 0 0 0 1 2 2 2
  spline S245 degree 2 poles (54.7617, 12.0517) (54.6686, 12.1) (54.5376, 12.1448) (54.4996, 12.1448) knots 0 0 0 1 2 2 2
  spline S246 degree 2 poles (54.4996, 12.1448) (54.1134, 12.1448) (53.5583, 11.5207) (53.5583, 11.1103) knots 0 0 0 1 2 2 2
  spline S247 degree 2 poles (53.5583, 11.1103) (53.5583, 10.7069) (53.8445, 10.3) (54.1341, 10.3) knots 0 0 0 1 2 2 2
  spline S248 degree 2 poles (54.1341, 10.3) (54.3686, 10.3) (54.5341, 10.3862) knots 0 0 0 1 1 1
  spline S249 degree 2 poles (54.5341, 10.3862) (54.6238, 10.4345) (54.7859, 10.5759) knots 0 0 0 1 1 1
  spline S250 degree 2 poles (54.7859, 10.5759) (54.7065, 11.231) (54.7065, 11.5552) knots 0 0 0 1 1 1
  spline S251 degree 2 poles (57.779, 9.8241) (57.5686, 9.8241) (57.541, 10.0552) knots 0 0 0 1 1 1
  line L51 (57.541, 10.0552) -> (57.4721, 10.6)
  spline S252 degree 2 poles (57.4721, 10.6) (57.4376, 10.8897) (57.4376, 11.1414) knots 0 0 0 1 1 1
  spline S253 degree 2 poles (57.4376, 11.1414) (57.4376, 11.2103) (57.4548, 11.5414) (57.4548, 11.6103) knots 0 0 0 1 2 2 2
  spline S254 degree 2 poles (57.4548, 11.6103) (57.4548, 12.1448) (57.2583, 12.1448) knots 0 0 0 1 1 1
  spline S255 degree 2 poles (57.2583, 12.1448) (56.979, 12.1448) (56.7272, 11.8172) knots 0 0 0 1 1 1
  spline S256 degree 2 poles (56.7272, 11.8172) (56.4996, 11.5172) (56.3721, 11.0586) knots 0 0 0 1 1 1
  spline S257 degree 2 poles (56.3721, 11.0586) (56.3652, 10.9621) (56.3479, 10.8172) knots 0 0 0 1 1 1
  spline S258 degree 2 poles (56.3479, 10.8172) (56.3341, 10.6931) (56.3341, 10.5759) knots 0 0 0 1 1 1
  spline S259 degree 2 poles (56.3341, 10.5759) (56.3341, 10.5034) (56.3652, 10.2069) (56.3652, 10.131) knots 0 0 0 1 2 2 2
  spline S260 degree 2 poles (56.3652, 10.131) (56.3652, 10.0207) (56.2272, 9.8828) (56.1203, 9.8828) knots 0 0 0 1 2 2 2
  spline S261 degree 2 poles (56.1203, 9.8828) (56.0134, 9.8828) (55.879, 10.0207) (55.879, 10.131) knots 0 0 0 1 2 2 2
  spline S262 degree 2 poles (55.879, 10.131) (55.879, 10.2069) (55.8479, 10.5034) (55.8479, 10.5793) knots 0 0 0 1 2 2 2
  spline S263 degree 2 poles (55.8479, 10.5793) (55.8479, 10.8345) (55.9169, 11.7345) (55.9169, 11.9897) knots 0 0 0 1 2 2 2
  spline S264 degree 2 poles (55.9169, 11.9897) (55.9169, 12.069) (55.8996, 12.3828) (55.8996, 12.4621) knots 0 0 0 1 2 2 2
  spline S265 degree 2 poles (55.8996, 12.4621) (55.8996, 12.569) (56.041, 12.7034) (56.1445, 12.7034) knots 0 0 0 1 2 2 2
  spline S266 degree 2 poles (56.1445, 12.7034) (56.3721, 12.7034) (56.3962, 12.3793) knots 0 0 0 1 1 1
  line L52 (56.3962, 12.3793) -> (56.4031, 12.0897)
  spline S267 degree 2 poles (56.4031, 12.0897) (56.8169, 12.6448) (57.2548, 12.6448) knots 0 0 0 1 1 1
  spline S268 degree 2 poles (57.2548, 12.6448) (57.6514, 12.6448) (57.8065, 12.2966) knots 0 0 0 1 1 1
  spline S269 degree 2 poles (57.8065, 12.2966) (57.9134, 12.0621) (57.9238, 11.6069) knots 0 0 0 1 1 1
  line L53 (57.9238, 11.6069) -> (57.9238, 11.3586)
  line L54 (57.9238, 11.3586) -> (57.9203, 11.1276)
  spline S270 degree 2 poles (57.9203, 11.1276) (57.9203, 10.9241) (58.0272, 10.2724) (58.0272, 10.069) knots 0 0 0 1 2 2 2
  spline S271 degree 2 poles (58.0272, 10.069) (58.0272, 9.9586) (57.8859, 9.8241) (57.779, 9.8241) knots 0 0 0 1 2 2 2
  spline S272 degree 2 poles (60.1893, 12.1069) (60.1376, 12.1069) (59.9962, 12.1172) (59.9445, 12.1172) knots 0 0 0 1 2 2 2
  spline S273 degree 2 poles (59.9445, 12.1172) (59.8859, 12.1172) (59.6065, 12.0793) knots 0 0 0 1 1 1
  line L55 (59.6065, 12.0793) -> (59.6514, 10.6172)
  line L56 (59.6514, 10.6172) -> (59.6548, 10.5103)
  line L57 (59.6548, 10.5103) -> (59.6583, 10.3828)
  spline S274 degree 2 poles (59.6583, 10.3828) (59.6686, 9.8414) (59.3996, 9.8414) knots 0 0 0 1 1 1
  spline S275 degree 2 poles (59.3996, 9.8414) (59.2996, 9.8414) (59.1548, 9.969) (59.1548, 10.0655) knots 0 0 0 1 2 2 2
  spline S276 degree 2 poles (59.1548, 10.0655) (59.1548, 10.1621) (59.1686, 10.5379) (59.1686, 10.631) knots 0 0 0 1 2 2 2
  line L58 (59.1686, 10.631) -> (59.1203, 12.0759)
  spline S277 degree 2 poles (59.1203, 12.0759) (58.941, 12.0828) (58.5721, 12.1172) knots 0 0 0 1 1 1
  spline S278 degree 2 poles (58.5721, 12.1172) (58.3514, 12.1483) (58.3514, 12.3621) knots 0 0 0 1 1 1
  spline S279 degree 2 poles (58.3514, 12.3621) (58.3514, 12.4724) (58.4859, 12.6138) (58.5893, 12.6138) knots 0 0 0 1 2 2 2
  line L59 (58.5893, 12.6138) -> (59.1065, 12.5724)
  spline S280 degree 2 poles (59.1065, 12.5724) (59.1065, 12.7) (59.0859, 13.1207) (59.0859, 13.2138) knots 0 0 0 1 2 2 2
  spline S281 degree 2 poles (59.0859, 13.2138) (59.0859, 13.3207) (59.2272, 13.4552) (59.3307, 13.4552) knots 0 0 0 1 2 2 2
  spline S282 degree 2 poles (59.3307, 13.4552) (59.5548, 13.4552) (59.5927, 13.0931) knots 0 0 0 1 1 1
  spline S283 degree 2 poles (59.5927, 13.0931) (59.5996, 13) (59.5996, 12.8724) knots 0 0 0 1 1 1
  line L60 (59.5996, 12.8724) -> (59.5962, 12.7276)
  line L61 (59.5962, 12.7276) -> (59.5927, 12.5759)
  spline S284 degree 2 poles (59.5927, 12.5759) (59.8996, 12.6138) (59.9445, 12.6138) knots 0 0 0 1 1 1
  spline S285 degree 2 poles (59.9445, 12.6138) (60.1996, 12.6138) (60.279, 12.5897) knots 0 0 0 1 1 1
  spline S286 degree 2 poles (60.279, 12.5897) (60.4307, 12.5414) (60.4307, 12.3586) knots 0 0 0 1 1 1
  spline S287 degree 2 poles (60.4307, 12.3586) (60.4307, 12.2483) (60.2962, 12.1069) (60.1893, 12.1069) knots 0 0 0 1 2 2 2
  spline S288 degree 2 poles (62.8514, 9.8345) (62.8065, 9.8345) (62.6824, 9.9448) knots 0 0 0 1 1 1
  spline S289 degree 2 poles (62.6824, 9.9448) (62.5721, 10.0448) (62.5169, 10.1241) knots 0 0 0 1 1 1
  spline S290 degree 2 poles (62.5169, 10.1241) (62.279, 9.9966) (61.9169, 9.8655) (61.7962, 9.8655) knots 0 0 0 1 2 2 2
  spline S291 degree 2 poles (61.7962, 9.8655) (61.2169, 9.8655) (60.9514, 10.1931) knots 0 0 0 1 1 1
  spline S292 degree 2 poles (60.9514, 10.1931) (60.7031, 10.5) (60.7031, 11.131) knots 0 0 0 1 1 1
  spline S293 degree 2 poles (60.7031, 11.131) (60.7031, 11.731) (61.5272, 12.5828) (62.0996, 12.5828) knots 0 0 0 1 2 2 2
  spline S294 degree 2 poles (62.0996, 12.5828) (62.3134, 12.5828) (62.5824, 12.4724) knots 0 0 0 1 1 1
  spline S295 degree 2 poles (62.5824, 12.4724) (62.9169, 12.331) (62.9169, 12.1379) knots 0 0 0 1 1 1
  spline S296 degree 2 poles (62.9169, 12.1379) (62.9169, 12.069) (62.8686, 12.0172) knots 0 0 0 1 1 1
  spline S297 degree 2 poles (62.8686, 12.0172) (62.8445, 11.9241) (62.8169, 11.4931) (62.8134, 11.1552) knots 0 0 0 1 2 2 2
  spline S298 degree 2 poles (62.8134, 11.1552) (62.81, 10.8483) (62.8548, 10.6724) knots 0 0 0 1 1 1
  spline S299 degree 2 poles (62.8548, 10.6724) (62.879, 10.5621) (63.01, 10.2345) knots 0 0 0 1 1 1
  spline S300 degree 2 poles (63.01, 10.2345) (63.0272, 10.1897) (63.0686, 10.1034) knots 0 0 0 1 1 1
  line L62 (63.0686, 10.1034) -> (63.0824, 10.0621)
  spline S301 degree 2 poles (63.0824, 10.0621) (63.0824, 9.9621) (62.9445, 9.8345) (62.8514, 9.8345) knots 0 0 0 1 2 2 2
  spline S302 degree 2 poles (62.3376, 11.5552) (62.3376, 11.6621) (62.3652, 11.9138) (62.3927, 12.0517) knots 0 0 0 1 2 2 2
  spline S303 degree 2 poles (62.3927, 12.0517) (62.2996, 12.1) (62.1686, 12.1448) (62.1307, 12.1448) knots 0 0 0 1 2 2 2
  spline S304 degree 2 poles (62.1307, 12.1448) (61.7445, 12.1448) (61.1893, 11.5207) (61.1893, 11.1103) knots 0 0 0 1 2 2 2
  spline S305 degree 2 poles (61.1893, 11.1103) (61.1893, 10.7069) (61.4755, 10.3) (61.7652, 10.3) knots 0 0 0 1 2 2 2
  spline S306 degree 2 poles (61.7652, 10.3) (61.9996, 10.3) (62.1652, 10.3862) knots 0 0 0 1 1 1
  spline S307 degree 2 poles (62.1652, 10.3862) (62.2548, 10.4345) (62.4169, 10.5759) knots 0 0 0 1 1 1
  spline S308 degree 2 poles (62.4169, 10.5759) (62.3376, 11.231) (62.3376, 11.5552) knots 0 0 0 1 1 1
  line L63 (64.141, 11.9448) -> (64.1065, 10.7138)
  spline S309 degree 2 poles (64.1065, 10.7138) (64.1065, 10.5172) (64.0859, 10.1414) knots 0 0 0 1 1 1
  spline S310 degree 2 poles (64.0859, 10.1414) (64.0617, 9.8931) (63.8445, 9.8931) knots 0 0 0 1 1 1
  spline S311 degree 2 poles (63.8445, 9.8931) (63.5996, 9.8931) (63.5996, 10.1448) knots 0 0 0 1 1 1
  spline S312 degree 2 poles (63.5996, 10.1448) (63.5996, 10.4448) (63.6548, 11.6448) (63.6548, 11.9448) knots 0 0 0 1 2 2 2
  spline S313 degree 2 poles (63.6548, 11.9448) (63.6548, 12.3345) (63.679, 13.3414) (63.679, 13.731) knots 0 0 0 1 2 2 2
  spline S314 degree 2 poles (63.679, 13.731) (63.679, 13.9793) (63.9203, 13.9793) knots 0 0 0 1 1 1
  spline S315 degree 2 poles (63.9203, 13.9793) (64.1652, 13.9793) (64.1652, 13.731) knots 0 0 0 1 1 1
  spline S316 degree 2 poles (64.1652, 13.731) (64.1652, 13.3414) (64.141, 12.3345) (64.141, 11.9448) knots 0 0 0 1 2 2 2
  spline S317 degree 2 poles (65.8307, 9.8552) (65.4169, 9.8552) (65.1169, 10.1621) knots 0 0 0 1 1 1
  spline S318 degree 2 poles (65.1169, 10.1621) (64.7824, 10.5034) (64.7652, 11.0793) knots 0 0 0 1 1 1
  spline S319 degree 2 poles (64.7652, 11.0793) (64.7514, 11.6379) (65.0479, 12.0621) knots 0 0 0 1 1 1
  spline S320 degree 2 poles (65.0479, 12.0621) (65.3927, 12.5655) (66.01, 12.5655) knots 0 0 0 1 1 1
  spline S321 degree 2 poles (66.01, 12.5655) (66.5065, 12.5655) (66.7583, 12.1138) knots 0 0 0 1 1 1
  spline S322 degree 2 poles (66.7583, 12.1138) (66.9617, 11.7483) (66.9548, 11.231) knots 0 0 0 1 1 1
  spline S323 degree 2 poles (66.9548, 11.231) (66.9479, 10.6828) (66.6686, 10.2966) knots 0 0 0 1 1 1
  spline S324 degree 2 poles (66.6686, 10.2966) (66.3514, 9.8552) (65.8307, 9.8552) knots 0 0 0 1 1 1
  spline S325 degree 2 poles (65.979, 12.0621) (65.6169, 12.0655) (65.4134, 11.7172) knots 0 0 0 1 1 1
  spline S326 degree 2 poles (65.4134, 11.7172) (65.2514, 11.4379) (65.2514, 11.0793) knots 0 0 0 1 1 1
  spline S327 degree 2 poles (65.2514, 11.0793) (65.2514, 10.7207) (65.4479, 10.5207) knots 0 0 0 1 1 1
  spline S328 degree 2 poles (65.4479, 10.5207) (65.61, 10.3552) (65.8307, 10.3552) knots 0 0 0 1 1 1
  spline S329 degree 2 poles (65.8307, 10.3552) (66.0893, 10.3552) (66.2721, 10.5414) knots 0 0 0 1 1 1
  spline S330 degree 2 poles (66.2721, 10.5414) (66.4824, 10.7517) (66.4962, 11.1034) knots 0 0 0 1 1 1
  spline S331 degree 2 poles (66.4962, 11.1034) (66.5307, 12.0586) (65.979, 12.0621) knots 0 0 0 1 1 1
  spline S332 degree 2 poles (68.7203, 9.8966) (68.341, 9.8966) (68.0341, 10.0448) knots 0 0 0 1 1 1
  spline S333 degree 2 poles (68.0341, 10.0448) (67.9548, 9.9276) (67.841, 9.9276) knots 0 0 0 1 1 1
  spline S334 degree 2 poles (67.841, 9.9276) (67.7445, 9.9276) (67.6134, 10.0586) (67.6134, 10.1586) knots 0 0 0 1 2 2 2
  spline S335 degree 2 poles (67.6134, 10.1586) (67.6134, 10.2207) (67.6272, 10.4724) (67.6272, 10.5379) knots 0 0 0 1 2 2 2
  spline S336 degree 2 poles (67.6272, 10.5379) (67.6272, 10.8) (67.5996, 11.8483) (67.5996, 12.1103) knots 0 0 0 1 2 2 2
  spline S337 degree 2 poles (67.5996, 12.1103) (67.5996, 12.2897) (67.6065, 13.2966) (67.6065, 13.4793) knots 0 0 0 1 2 2 2
  spline S338 degree 2 poles (67.6065, 13.4793) (67.6065, 13.6276) (67.6686, 13.7448) knots 0 0 0 1 1 1
  spline S339 degree 2 poles (67.6686, 13.7448) (67.7479, 13.8966) (67.8927, 13.8966) knots 0 0 0 1 1 1
  spline S340 degree 2 poles (67.8927, 13.8966) (68.079, 13.8966) (68.079, 13.6828) knots 0 0 0 1 1 1
  spline S341 degree 2 poles (68.079, 13.6828) (68.079, 13.6448) (68.0548, 13.5138) (68.0548, 13.4793) knots 0 0 0 1 2 2 2
  line L64 (68.0548, 13.4793) -> (68.0445, 12.9345)
  line L65 (68.0445, 12.9345) -> (68.041, 12.3034)
  spline S342 degree 2 poles (68.041, 12.3034) (68.2548, 12.4517) (68.6445, 12.5966) (68.8134, 12.5966) knots 0 0 0 1 2 2 2
  spline S343 degree 2 poles (68.8134, 12.5966) (69.3479, 12.5966) (69.679, 12.1897) knots 0 0 0 1 1 1
  spline S344 degree 2 poles (69.679, 12.1897) (69.9893, 11.8069) (69.9893, 11.2483) knots 0 0 0 1 1 1
  spline S345 degree 2 poles (69.9893, 11.2483) (69.9893, 10.6828) (69.2617, 9.8966) (68.7203, 9.8966) knots 0 0 0 1 2 2 2
  spline S346 degree 2 poles (68.8134, 12.1276) (68.6134, 12.1276) (68.3996, 12.0138) knots 0 0 0 1 1 1
  spline S347 degree 2 poles (68.3996, 12.0138) (68.2962, 11.9586) (68.0445, 11.769) knots 0 0 0 1 1 1
  line L66 (68.0445, 11.769) -> (68.041, 11.3414)
  line L67 (68.041, 11.3414) -> (68.041, 10.9552)
  line L68 (68.041, 10.9552) -> (68.0445, 10.5517)
  spline S348 degree 2 poles (68.0445, 10.5517) (68.1617, 10.4966) (68.379, 10.4138) knots 0 0 0 1 1 1
  spline S349 degree 2 poles (68.379, 10.4138) (68.5307, 10.3655) (68.7203, 10.3655) knots 0 0 0 1 1 1
  spline S350 degree 2 poles (68.7203, 10.3655) (69.079, 10.3655) (69.5376, 10.869) (69.5376, 11.2448) knots 0 0 0 1 2 2 2
  spline S351 degree 2 poles (69.5376, 11.2448) (69.5376, 11.6138) (69.3514, 11.8621) knots 0 0 0 1 1 1
  spline S352 degree 2 poles (69.3514, 11.8621) (69.1514, 12.1276) (68.8134, 12.1276) knots 0 0 0 1 1 1
  spline S353 degree 2 poles (72.5031, 9.8345) (72.4583, 9.8345) (72.3341, 9.9448) knots 0 0 0 1 1 1
  spline S354 degree 2 poles (72.3341, 9.9448) (72.2238, 10.0448) (72.1686, 10.1241) knots 0 0 0 1 1 1
  spline S355 degree 2 poles (72.1686, 10.1241) (71.9307, 9.9966) (71.5686, 9.8655) (71.4479, 9.8655) knots 0 0 0 1 2 2 2
  spline S356 degree 2 poles (71.4479, 9.8655) (70.8686, 9.8655) (70.6031, 10.1931) knots 0 0 0 1 1 1
  spline S357 degree 2 poles (70.6031, 10.1931) (70.3548, 10.5) (70.3548, 11.131) knots 0 0 0 1 1 1
  spline S358 degree 2 poles (70.3548, 11.131) (70.3548, 11.731) (71.179, 12.5828) (71.7514, 12.5828) knots 0 0 0 1 2 2 2
  spline S359 degree 2 poles (71.7514, 12.5828) (71.9652, 12.5828) (72.2341, 12.4724) knots 0 0 0 1 1 1
  spline S360 degree 2 poles (72.2341, 12.4724) (72.5686, 12.331) (72.5686, 12.1379) knots 0 0 0 1 1 1
  spline S361 degree 2 poles (72.5686, 12.1379) (72.5686, 12.069) (72.5203, 12.0172) knots 0 0 0 1 1 1
  spline S362 degree 2 poles (72.5203, 12.0172) (72.4962, 11.9241) (72.4686, 11.4931) (72.4652, 11.1552) knots 0 0 0 1 2 2 2
  spline S363 degree 2 poles (72.4652, 11.1552) (72.4617, 10.8483) (72.5065, 10.6724) knots 0 0 0 1 1 1
  spline S364 degree 2 poles (72.5065, 10.6724) (72.5307, 10.5621) (72.6617, 10.2345) knots 0 0 0 1 1 1
  spline S365 degree 2 poles (72.6617, 10.2345) (72.679, 10.1897) (72.7203, 10.1034) knots 0 0 0 1 1 1
  line L69 (72.7203, 10.1034) -> (72.7341, 10.0621)
  spline S366 degree 2 poles (72.7341, 10.0621) (72.7341, 9.9621) (72.5962, 9.8345) (72.5031, 9.8345) knots 0 0 0 1 2 2 2
  spline S367 degree 2 poles (71.9893, 11.5552) (71.9893, 11.6621) (72.0169, 11.9138) (72.0445, 12.0517) knots 0 0 0 1 2 2 2
  spline S368 degree 2 poles (72.0445, 12.0517) (71.9514, 12.1) (71.8203, 12.1448) (71.7824, 12.1448) knots 0 0 0 1 2 2 2
  spline S369 degree 2 poles (71.7824, 12.1448) (71.3962, 12.1448) (70.841, 11.5207) (70.841, 11.1103) knots 0 0 0 1 2 2 2
  spline S370 degree 2 poles (70.841, 11.1103) (70.841, 10.7069) (71.1272, 10.3) (71.4169, 10.3) knots 0 0 0 1 2 2 2
  spline S371 degree 2 poles (71.4169, 10.3) (71.6514, 10.3) (71.8169, 10.3862) knots 0 0 0 1 1 1
  spline S372 degree 2 poles (71.8169, 10.3862) (71.9065, 10.4345) (72.0686, 10.5759) knots 0 0 0 1 1 1